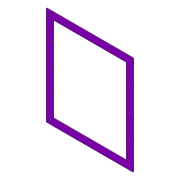
# Autodesk Inventor part: enclosureFloorFlange
Saved by Autodesk Inventor 2017 (Build 210142000, 142)
## iProperties
Created: 2016-11-30
Part Number: enclosureFloorFlange
Material: Generic
Document SubType Name: Modeling
Designer: krosie
Density: 1 g/cm^3
Appearance: Default
Author: krosie
Autodesk Inventor part; units mm, degrees
ref_plane "YZ Plane" through (0, 0, 0) normal (1, 0, 0) x (0, 1, 0)
ref_plane "XZ Plane" through (0, 0, 0) normal (0, 1, 0) x (-1, 0, 0)
ref_plane "XY Plane" through (0, 0, 0) normal (0, 0, 1) x (1, 0, 0)
sketch "Sketch1" plane through (0, 0, 0) normal (0, 1, 0) x (-1, 0, 0)
  line L0 (-363.3, 419.1) -> (363.3, 419.1)
  line L1 (368.3, 414.1) -> (368.3, -414.1)
  line L2 (363.3, -419.1) -> (-363.3, -419.1)
  line L3 (-368.3, -414.1) -> (-368.3, 414.1)
  line L4 (-368.3, 419.1) -> (368.3, -419.1) construction
  line L5 (368.3, 419.1) -> (-368.3, -419.1) construction
  line L6 (303.3, 359.1) -> (-303.3, 359.1)
  line L7 (-308.3, 354.1) -> (-308.3, -354.1)
  line L8 (-303.3, -359.1) -> (303.3, -359.1)
  line L9 (308.3, -354.1) -> (308.3, 354.1)
  arc A0 (308.3, 354.1) -> (303.3, 359.1) centre (303.3, 354.1) ccw
  arc A1 (303.3, -359.1) -> (308.3, -354.1) centre (303.3, -354.1) ccw
  arc A2 (-303.3, 359.1) -> (-308.3, 354.1) centre (-303.3, 354.1) ccw
  arc A3 (-308.3, -354.1) -> (-303.3, -359.1) centre (-303.3, -354.1) ccw
  arc A4 (368.3, 414.1) -> (363.3, 419.1) centre (363.3, 414.1) ccw
  arc A5 (-363.3, 419.1) -> (-368.3, 414.1) centre (-363.3, 414.1) ccw
  arc A6 (-368.3, -414.1) -> (-363.3, -419.1) centre (-363.3, -414.1) ccw
  arc A7 (363.3, -419.1) -> (368.3, -414.1) centre (363.3, -414.1) ccw
  point P0 (0, 0)
  dimension "d0" = 736.6
  dimension "d1" = 838.2
  dimension "d2" = 60
  dimension "d4" = 5
  constraints: 20 end point, 16 point on circle, 16 tangent, 8 centre point, 8 point on line, 7 equal radius, 4 parallel, 2 midpoint, 2 perpendicular, 1 horizontal, 3 other
  measures "d0" distance of L4.end L5.end
  measures "d1" distance of L5.start L4.end
  measures "d2" distance between parallel lines of L0 L6
  measures "d4" radius of A0
extrude "Extrusion1" add sketch "Sketch1" along normal blind 5
sketch "Sketch2" plane through (0, 5, 0) normal (0, 1, 0) x (1, 0, 0)
  circle A0 centre (-334, 384.8) radius 6 projected
  circle A1 centre (-250.5, 384.8) radius 6 projected
  circle A2 centre (-167, 384.8) radius 6 projected
  circle A3 centre (-83.5, 384.8) radius 6 projected
  circle A4 centre (0, 384.8) radius 6 projected
  circle A5 centre (83.5, 384.8) radius 6 projected
  circle A6 centre (-334, 288.6) radius 6 projected
  circle A7 centre (-334, 96.2) radius 6 projected
  circle A8 centre (-334, -96.2) radius 6 projected
  circle A9 centre (-334, -192.4) radius 6 projected
  circle A10 centre (-334, -288.6) radius 6 projected
  circle A11 centre (-334, -384.8) radius 6 projected
  circle A12 centre (-334, 0) radius 6 projected
  circle A13 centre (-334, 192.4) radius 6 projected
  circle A14 centre (-250.5, -384.8) radius 6 projected
  circle A15 centre (-167, -384.8) radius 6 projected
  circle A16 centre (-83.5, -384.8) radius 6 projected
  circle A17 centre (0, -384.8) radius 6 projected
  circle A18 centre (83.5, -384.8) radius 6 projected
  circle A19 centre (167, -384.8) radius 6 projected
  circle A20 centre (250.5, -384.8) radius 6 projected
  circle A21 centre (334, -384.8) radius 6 projected
  circle A22 centre (334, -288.6) radius 6 projected
  circle A23 centre (334, -192.4) radius 6 projected
  circle A24 centre (334, -96.2) radius 6 projected
  circle A25 centre (334, 0) radius 6 projected
  circle A26 centre (334, 96.2) radius 6 projected
  circle A27 centre (334, 192.4) radius 6 projected
  circle A28 centre (334, 288.6) radius 6 projected
  circle A29 centre (334, 384.8) radius 6 projected
  circle A30 centre (167, 384.8) radius 6 projected
  circle A31 centre (250.5, 384.8) radius 6 projected
  point P0 (0, 0)
extrude "Extrusion2" cut sketch "Sketch2" against normal up to next contours A0 | A2 | A4 | A9 | A11 | A12 | A13 | A15 | A17 | A19 | A21 | A23 | A25 | A27 | A29 | A30
body "Solid1"
